Autodesk Inventor part; units mm, degrees
(part 2 of 3)
  line L293 (-765.7551, -84.2338) -> (-765.6693, -83.5816) projected
  line L294 (-765.6693, -83.5816) -> (-765.4175, -82.9738) projected
  line L295 (-765.4175, -82.9738) -> (-765.017, -82.4519) projected
  line L296 (-765.017, -82.4519) -> (-764.4951, -82.0514) projected
  line L297 (-764.4951, -82.0514) -> (-763.8874, -81.7997) projected
  line L298 (-763.8874, -81.7997) -> (-763.2351, -81.7138) projected
  line L299 (-763.2351, -81.7138) -> (-762.5829, -81.7997) projected
  line L300 (-762.5829, -81.7997) -> (-761.9751, -82.0514) projected
  line L301 (-761.9751, -82.0514) -> (-761.4532, -82.4519) projected
  line L302 (-761.4532, -82.4519) -> (-761.0528, -82.9738) projected
  line L303 (-691.0528, -27.9738) -> (-690.801, -28.5816) projected
  line L304 (-690.801, -28.5816) -> (-690.7151, -29.2338) projected
  line L305 (-690.7151, -29.2338) -> (-690.801, -29.886) projected
  line L306 (-690.801, -29.886) -> (-691.0528, -30.4938) projected
  line L307 (-691.0528, -30.4938) -> (-691.4532, -31.0157) projected
  line L308 (-691.4532, -31.0157) -> (-691.9751, -31.4162) projected
  line L309 (-691.9751, -31.4162) -> (-692.5829, -31.6679) projected
  line L310 (-692.5829, -31.6679) -> (-693.2351, -31.7538) projected
  line L311 (-693.2351, -31.7538) -> (-693.8874, -31.6679) projected
  line L312 (-693.8874, -31.6679) -> (-694.4951, -31.4162) projected
  line L313 (-694.4951, -31.4162) -> (-695.0171, -31.0157) projected
  line L314 (-695.0171, -31.0157) -> (-695.4175, -30.4938) projected
  line L315 (-695.4175, -30.4938) -> (-695.6693, -29.886) projected
  line L316 (-695.6693, -29.886) -> (-695.7551, -29.2338) projected
  line L317 (-695.7551, -29.2338) -> (-695.6693, -28.5816) projected
  line L318 (-695.6693, -28.5816) -> (-695.4175, -27.9738) projected
  line L319 (-695.4175, -27.9738) -> (-695.0171, -27.4519) projected
  line L320 (-695.0171, -27.4519) -> (-694.4951, -27.0514) projected
  line L321 (-694.4951, -27.0514) -> (-693.8874, -26.7997) projected
  line L322 (-693.8874, -26.7997) -> (-693.2351, -26.7138) projected
  line L323 (-693.2351, -26.7138) -> (-692.5829, -26.7997) projected
  line L324 (-692.5829, -26.7997) -> (-691.9751, -27.0514) projected
  line L325 (-691.9751, -27.0514) -> (-691.4532, -27.4519) projected
  line L326 (-691.4532, -27.4519) -> (-691.0528, -27.9738) projected
  line L327 (-691.0528, -660.4938) -> (-691.4532, -661.0157) projected
  line L328 (-691.4532, -661.0157) -> (-691.9751, -661.4162) projected
  line L329 (-691.9751, -661.4162) -> (-692.5829, -661.6679) projected
  line L330 (-692.5829, -661.6679) -> (-693.2351, -661.7538) projected
  line L331 (-693.2351, -661.7538) -> (-693.8874, -661.6679) projected
  line L332 (-693.8874, -661.6679) -> (-694.4951, -661.4162) projected
  line L333 (-694.4951, -661.4162) -> (-695.0171, -661.0157) projected
  line L334 (-695.0171, -661.0157) -> (-695.4175, -660.4938) projected
  line L335 (-695.4175, -660.4938) -> (-695.6693, -659.886) projected
  line L336 (-695.6693, -659.886) -> (-695.7551, -659.2338) projected
  line L337 (-695.7551, -659.2338) -> (-695.6693, -658.5816) projected
  line L338 (-695.6693, -658.5816) -> (-695.4175, -657.9738) projected
  line L339 (-695.4175, -657.9738) -> (-695.0171, -657.4519) projected
  line L340 (-695.0171, -657.4519) -> (-694.4951, -657.0514) projected
  line L341 (-694.4951, -657.0514) -> (-693.8874, -656.7997) projected
  line L342 (-693.8874, -656.7997) -> (-693.2351, -656.7138) projected
  line L343 (-693.2351, -656.7138) -> (-692.5829, -656.7997) projected
  line L344 (-692.5829, -656.7997) -> (-691.9751, -657.0514) projected
  line L345 (-691.9751, -657.0514) -> (-691.4532, -657.4519) projected
  line L346 (-691.4532, -657.4519) -> (-691.0528, -657.9738) projected
  line L347 (-691.0528, -657.9738) -> (-690.801, -658.5816) projected
  line L348 (-690.801, -658.5816) -> (-690.7151, -659.2338) projected
  line L349 (-690.7151, -659.2338) -> (-690.801, -659.886) projected
  line L350 (-690.801, -659.886) -> (-691.0528, -660.4938) projected
  line L351 (-761.0528, -27.9738) -> (-760.801, -28.5816) projected
  line L352 (-760.801, -28.5816) -> (-760.7151, -29.2338) projected
  line L353 (-760.7151, -29.2338) -> (-760.801, -29.886) projected
  line L354 (-760.801, -29.886) -> (-761.0528, -30.4938) projected
  line L355 (-761.0528, -30.4938) -> (-761.4532, -31.0157) projected
  line L356 (-761.4532, -31.0157) -> (-761.9751, -31.4162) projected
  line L357 (-761.9751, -31.4162) -> (-762.5829, -31.6679) projected
  line L358 (-762.5829, -31.6679) -> (-763.2351, -31.7538) projected
  line L359 (-763.2351, -31.7538) -> (-763.8874, -31.6679) projected
  line L360 (-763.8874, -31.6679) -> (-764.4951, -31.4162) projected
  line L361 (-764.4951, -31.4162) -> (-765.017, -31.0157) projected
  line L362 (-765.017, -31.0157) -> (-765.4175, -30.4938) projected
  line L363 (-765.4175, -30.4938) -> (-765.6693, -29.886) projected
  line L364 (-765.6693, -29.886) -> (-765.7551, -29.2338) projected
  line L365 (-765.7551, -29.2338) -> (-765.6693, -28.5816) projected
  line L366 (-765.6693, -28.5816) -> (-765.4175, -27.9738) projected
  line L367 (-765.4175, -27.9738) -> (-765.017, -27.4519) projected
  line L368 (-765.017, -27.4519) -> (-764.4951, -27.0514) projected
  line L369 (-764.4951, -27.0514) -> (-763.8874, -26.7997) projected
  line L370 (-763.8874, -26.7997) -> (-763.2351, -26.7138) projected
  line L371 (-763.2351, -26.7138) -> (-762.5829, -26.7997) projected
  line L372 (-762.5829, -26.7997) -> (-761.9751, -27.0514) projected
  line L373 (-761.9751, -27.0514) -> (-761.4532, -27.4519) projected
  line L374 (-761.4532, -27.4519) -> (-761.0528, -27.9738) projected
  line L375 (-761.0528, -657.9738) -> (-760.801, -658.5816) projected
  line L376 (-760.801, -658.5816) -> (-760.7151, -659.2338) projected
  line L377 (-760.7151, -659.2338) -> (-760.801, -659.886) projected
  line L378 (-760.801, -659.886) -> (-761.0528, -660.4938) projected
  line L379 (-761.0528, -660.4938) -> (-761.4532, -661.0157) projected
  line L380 (-761.4532, -661.0157) -> (-761.9751, -661.4162) projected
  line L381 (-761.9751, -661.4162) -> (-762.5829, -661.6679) projected
  line L382 (-762.5829, -661.6679) -> (-763.2351, -661.7538) projected
  line L383 (-763.2351, -661.7538) -> (-763.8874, -661.6679) projected
  line L384 (-763.8874, -661.6679) -> (-764.4951, -661.4162) projected
  line L385 (-764.4951, -661.4162) -> (-765.017, -661.0157) projected
  line L386 (-765.017, -661.0157) -> (-765.4175, -660.4938) projected
  line L387 (-765.4175, -660.4938) -> (-765.6693, -659.886) projected
  line L388 (-765.6693, -659.886) -> (-765.7551, -659.2338) projected
  line L389 (-765.7551, -659.2338) -> (-765.6693, -658.5816) projected
  line L390 (-765.6693, -658.5816) -> (-765.4175, -657.9738) projected
  line L391 (-765.4175, -657.9738) -> (-765.017, -657.4519) projected
  line L392 (-765.017, -657.4519) -> (-764.4951, -657.0514) projected
  line L393 (-764.4951, -657.0514) -> (-763.8874, -656.7997) projected
  line L394 (-763.8874, -656.7997) -> (-763.2351, -656.7138) projected
  line L395 (-763.2351, -656.7138) -> (-762.5829, -656.7997) projected
  line L396 (-762.5829, -656.7997) -> (-761.9751, -657.0514) projected
  line L397 (-761.9751, -657.0514) -> (-761.4532, -657.4519) projected
  line L398 (-761.4532, -657.4519) -> (-761.0528, -657.9738) projected
  line L399 (-640.017, -661.0157) -> (-640.4175, -660.4938) projected
  line L400 (-640.4175, -660.4938) -> (-640.6693, -659.886) projected
  line L401 (-640.6693, -659.886) -> (-640.7551, -659.2338) projected
  line L402 (-640.7551, -659.2338) -> (-640.6693, -658.5816) projected
  line L403 (-640.6693, -658.5816) -> (-640.4175, -657.9738) projected
  line L404 (-640.4175, -657.9738) -> (-640.017, -657.4519) projected
  line L405 (-640.017, -657.4519) -> (-639.4951, -657.0514) projected
  line L406 (-639.4951, -657.0514) -> (-638.8874, -656.7997) projected
  line L407 (-638.8874, -656.7997) -> (-638.2351, -656.7138) projected
  line L408 (-638.2351, -656.7138) -> (-637.5829, -656.7997) projected
  line L409 (-637.5829, -656.7997) -> (-636.9751, -657.0514) projected
  line L410 (-636.9751, -657.0514) -> (-636.4532, -657.4519) projected
  line L411 (-636.4532, -657.4519) -> (-636.0528, -657.9738) projected
  line L412 (-636.0528, -657.9738) -> (-635.801, -658.5816) projected
  line L413 (-635.801, -658.5816) -> (-635.7152, -659.2338) projected
  line L414 (-635.7152, -659.2338) -> (-635.801, -659.886) projected
  line L415 (-635.801, -659.886) -> (-636.0528, -660.4938) projected
  line L416 (-636.0528, -660.4938) -> (-636.4532, -661.0157) projected
  line L417 (-636.4532, -661.0157) -> (-636.9751, -661.4162) projected
  line L418 (-636.9751, -661.4162) -> (-637.5829, -661.6679) projected
  line L419 (-637.5829, -661.6679) -> (-638.2351, -661.7538) projected
  line L420 (-638.2351, -661.7538) -> (-638.8874, -661.6679) projected
  line L421 (-638.8874, -661.6679) -> (-639.4951, -661.4162) projected
  line L422 (-639.4951, -661.4162) -> (-640.017, -661.0157) projected
  line L423 (-636.0528, -27.9738) -> (-635.801, -28.5816) projected
  line L424 (-635.801, -28.5816) -> (-635.7152, -29.2338) projected
  line L425 (-635.7152, -29.2338) -> (-635.801, -29.886) projected
  line L426 (-635.801, -29.886) -> (-636.0528, -30.4938) projected
  line L427 (-636.0528, -30.4938) -> (-636.4532, -31.0157) projected
  line L428 (-636.4532, -31.0157) -> (-636.9751, -31.4162) projected
  line L429 (-636.9751, -31.4162) -> (-637.5829, -31.6679) projected
  line L430 (-637.5829, -31.6679) -> (-638.2351, -31.7538) projected
  line L431 (-638.2351, -31.7538) -> (-638.8874, -31.6679) projected
  line L432 (-638.8874, -31.6679) -> (-639.4951, -31.4162) projected
  line L433 (-639.4951, -31.4162) -> (-640.017, -31.0157) projected
  line L434 (-640.017, -31.0157) -> (-640.4175, -30.4938) projected
  line L435 (-640.4175, -30.4938) -> (-640.6693, -29.886) projected
  line L436 (-640.6693, -29.886) -> (-640.7551, -29.2338) projected
  line L437 (-640.7551, -29.2338) -> (-640.6693, -28.5816) projected
  line L438 (-640.6693, -28.5816) -> (-640.4175, -27.9738) projected
  line L439 (-640.4175, -27.9738) -> (-640.017, -27.4519) projected
  line L440 (-640.017, -27.4519) -> (-639.4951, -27.0514) projected
  line L441 (-639.4951, -27.0514) -> (-638.8874, -26.7997) projected
  line L442 (-638.8874, -26.7997) -> (-638.2351, -26.7138) projected
  line L443 (-638.2351, -26.7138) -> (-637.5829, -26.7997) projected
  line L444 (-637.5829, -26.7997) -> (-636.9751, -27.0514) projected
  line L445 (-636.9751, -27.0514) -> (-636.4532, -27.4519) projected
  line L446 (-636.4532, -27.4519) -> (-636.0528, -27.9738) projected
  line L447 (-727.2351, -219.1338) -> (-726.821, -219.1883) projected
  line L448 (-726.821, -219.1883) -> (-726.4351, -219.3482) projected
  line L449 (-726.4351, -219.3482) -> (-726.1038, -219.6024) projected
  line L450 (-726.1038, -219.6024) -> (-725.8495, -219.9338) projected
  line L451 (-725.8495, -219.9338) -> (-725.6896, -220.3197) projected
  line L452 (-725.6896, -220.3197) -> (-725.6351, -220.7338) projected
  line L453 (-725.6351, -220.7338) -> (-725.6896, -221.1479) projected
  line L454 (-725.6896, -221.1479) -> (-725.8495, -221.5338) projected
  line L455 (-725.8495, -221.5338) -> (-726.1038, -221.8651) projected
  line L456 (-726.1038, -221.8651) -> (-726.4351, -222.1194) projected
  line L457 (-726.4351, -222.1194) -> (-726.821, -222.2793) projected
  line L458 (-726.821, -222.2793) -> (-727.2351, -222.3338) projected
  line L459 (-727.2351, -222.3338) -> (-727.6493, -222.2793) projected
  line L460 (-727.6493, -222.2793) -> (-728.0351, -222.1194) projected
  line L461 (-728.0351, -222.1194) -> (-728.3665, -221.8651) projected
  line L462 (-728.3665, -221.8651) -> (-728.6208, -221.5338) projected
  line L463 (-728.6208, -221.5338) -> (-728.7806, -221.1479) projected
  line L464 (-728.7806, -221.1479) -> (-728.8351, -220.7338) projected
  line L465 (-728.8351, -220.7338) -> (-728.7806, -220.3197) projected
  line L466 (-728.7806, -220.3197) -> (-728.6208, -219.9338) projected
  line L467 (-728.6208, -219.9338) -> (-728.3665, -219.6024) projected
  line L468 (-728.3665, -219.6024) -> (-728.0351, -219.3482) projected
  line L469 (-728.0351, -219.3482) -> (-727.6493, -219.1883) projected
  line L470 (-727.6493, -219.1883) -> (-727.2351, -219.1338) projected
  line L471 (-678.2351, -604.2338) -> (-611.7707, -670.6983) projected
  line L472 (-678.2351, -84.2338) -> (-678.2351, -604.2338) projected
  line L473 (-611.7707, -17.7693) -> (-678.2351, -84.2338) projected
  line L474 (-611.5131, -17.4555) -> (-611.7707, -17.7693) projected
  line L475 (-611.3217, -17.0974) -> (-611.5131, -17.4555) projected
  line L476 (-611.2039, -16.7089) -> (-611.3217, -17.0974) projected
  line L477 (-611.1641, -16.3049) -> (-611.2039, -16.7089) projected
  line L478 (-611.2039, -15.9008) -> (-611.1641, -16.3049) projected
  line L479 (-611.3217, -15.5123) -> (-611.2039, -15.9008) projected
  line L480 (-611.5131, -15.1542) -> (-611.3217, -15.5123) projected
  line L481 (-611.7707, -14.8404) -> (-611.5131, -15.1542) projected
  line L482 (-612.0845, -14.5828) -> (-611.7707, -14.8404) projected
  line L483 (-612.4426, -14.3915) -> (-612.0845, -14.5828) projected
  line L484 (-612.8311, -14.2736) -> (-612.4426, -14.3915) projected
  line L485 (-613.2351, -14.2338) -> (-612.8311, -14.2736) projected
  line L486 (-777.2351, -14.2338) -> (-613.2351, -14.2338) projected
  line L487 (-777.2351, -674.2338) -> (-777.2351, -14.2338) projected
  line L488 (-613.2351, -674.2338) -> (-777.2351, -674.2338) projected
  line L489 (-612.8311, -674.194) -> (-613.2351, -674.2338) projected
  line L490 (-612.4426, -674.0761) -> (-612.8311, -674.194) projected
  line L491 (-612.0845, -673.8848) -> (-612.4426, -674.0761) projected
  line L492 (-611.7707, -673.6272) -> (-612.0845, -673.8848) projected
  line L493 (-611.5131, -673.3134) -> (-611.7707, -673.6272) projected
  line L494 (-611.3217, -672.9553) -> (-611.5131, -673.3134) projected
  line L495 (-611.2039, -672.5668) -> (-611.3217, -672.9553) projected
  line L496 (-611.1641, -672.1627) -> (-611.2039, -672.5668) projected
  line L497 (-611.2039, -671.7587) -> (-611.1641, -672.1627) projected
  line L498 (-611.3217, -671.3702) -> (-611.2039, -671.7587) projected
  line L499 (-611.5131, -671.0121) -> (-611.3217, -671.3702) projected
  line L500 (-611.7707, -670.6983) -> (-611.5131, -671.0121) projected
  line L501 (-747.1924, -48.5812) -> (-747.2351, -49.2338)
  line L502 (-747.2351, -49.2338) -> (-747.2351, -210.2338)
  line L503 (-747.2351, -210.2338) -> (-747.1924, -210.8864)
  line L504 (-747.1924, -210.8864) -> (-747.0648, -211.5279)
  line L505 (-747.0648, -211.5279) -> (-746.8545, -212.1472)
  line L506 (-746.8545, -212.1472) -> (-746.5653, -212.7338)
  line L507 (-746.5653, -212.7338) -> (-746.2019, -213.2776)
  line L508 (-746.2019, -213.2776) -> (-745.7707, -213.7693)
  line L509 (-745.7707, -213.7693) -> (-745.2789, -214.2006)
  line L510 (-745.2789, -214.2006) -> (-744.7351, -214.5639)
  line L511 (-744.7351, -214.5639) -> (-744.1486, -214.8532)
  line L512 (-744.1486, -214.8532) -> (-743.5292, -215.0634)
  line L513 (-743.5292, -215.0634) -> (-742.8878, -215.191)
  line L514 (-742.8878, -215.191) -> (-742.2351, -215.2338)
  line L515 (-742.2351, -215.2338) -> (-713.2351, -215.2338)
  line L516 (-713.2351, -215.2338) -> (-712.5825, -215.191)
  line L517 (-712.5825, -215.191) -> (-711.941, -215.0634)
  line L518 (-711.941, -215.0634) -> (-711.3217, -214.8532)
  line L519 (-711.3217, -214.8532) -> (-710.7351, -214.5639)
  line L520 (-710.7351, -214.5639) -> (-710.1913, -214.2006)
  line L521 (-710.1913, -214.2006) -> (-709.6996, -213.7693)
  line L522 (-709.6996, -213.7693) -> (-709.2684, -213.2776)
  line L523 (-709.2684, -213.2776) -> (-708.905, -212.7338)
  line L524 (-708.905, -212.7338) -> (-708.6157, -212.1472)
  line L525 (-708.6157, -212.1472) -> (-708.4055, -211.5279)
  line L526 (-708.4055, -211.5279) -> (-708.2779, -210.8864)
  line L527 (-708.2779, -210.8864) -> (-708.2351, -210.2338)
  line L528 (-708.2351, -210.2338) -> (-708.2351, -49.2338)
  line L529 (-708.2351, -49.2338) -> (-708.2779, -48.5812)
  line L530 (-708.2779, -48.5812) -> (-708.4055, -47.9397)
  line L531 (-708.4055, -47.9397) -> (-708.6157, -47.3204)
  line L532 (-708.6157, -47.3204) -> (-708.905, -46.7338)
  line L533 (-708.905, -46.7338) -> (-709.2684, -46.19)
  line L534 (-709.2684, -46.19) -> (-709.6996, -45.6983)
  line L535 (-709.6996, -45.6983) -> (-710.1913, -45.267)
  line L536 (-710.1913, -45.267) -> (-710.7351, -44.9037)
  line L537 (-710.7351, -44.9037) -> (-711.3217, -44.6144)
  line L538 (-711.3217, -44.6144) -> (-711.941, -44.4042)
  line L539 (-711.941, -44.4042) -> (-712.5825, -44.2766)
  line L540 (-712.5825, -44.2766) -> (-713.2351, -44.2338)
  line L541 (-713.2351, -44.2338) -> (-742.2351, -44.2338)
  line L542 (-742.2351, -44.2338) -> (-742.8878, -44.2766)
  line L543 (-742.8878, -44.2766) -> (-743.5292, -44.4042)
  line L544 (-743.5292, -44.4042) -> (-744.1486, -44.6144)
  line L545 (-744.1486, -44.6144) -> (-744.7351, -44.9037)
  line L546 (-744.7351, -44.9037) -> (-745.2789, -45.267)
  line L547 (-745.2789, -45.267) -> (-745.7707, -45.6983)
  line L548 (-745.7707, -45.6983) -> (-746.2019, -46.19)
  line L549 (-746.2019, -46.19) -> (-746.5653, -46.7338)
  line L550 (-746.5653, -46.7338) -> (-746.8545, -47.3204)
  line L551 (-746.8545, -47.3204) -> (-747.0648, -47.9397)
  line L552 (-747.0648, -47.9397) -> (-747.1924, -48.5812)
  point P0 (-1999.0141, -29.8543)
  constraints: 210 end point, 52 symmetric about line, 1 horizontal, 1 midpoint
extrude "Extrusion2" cut sketch "Sketch2" against normal blind 3 contours L552 L551 L550 L549 L548 L547 L546 L545 L544 L543 L542 L541 L540 L539 L538 L537 L536 L535 L534 L533 L532 L531 L530 L529 L528 L527 L526 L525 L524 L523 L522 L521 L520 L519 L518 L517 L516 L515 L514 L513 L512 L511 L510 L509 L508 L507 L506 L505 L504 L503 L502 L501
sketch "Sketch3" plane through (-1999.0141, 29.8543, -2600.6334) normal (0, 0, -1) x (-1, 0, 0)
  line L0 (-746.2019, -213.2776) -> (-746.5653, -212.7338) projected
  line L1 (-746.5653, -212.7338) -> (-746.8545, -212.1472) projected
  line L2 (-746.8545, -212.1472) -> (-747.0648, -211.5279) projected
  line L3 (-747.0648, -211.5279) -> (-747.1924, -210.8864) projected
  line L4 (-747.1924, -210.8864) -> (-747.2351, -210.2338) projected
  line L5 (-747.2351, -210.2338) -> (-747.2351, -49.2338) projected
  line L6 (-747.2351, -49.2338) -> (-747.1924, -48.5812) projected
  line L7 (-747.1924, -48.5812) -> (-747.0648, -47.9397) projected
  line L8 (-747.0648, -47.9397) -> (-746.8545, -47.3204) projected
  line L9 (-746.8545, -47.3204) -> (-746.5653, -46.7338) projected
  line L10 (-746.5653, -46.7338) -> (-746.2019, -46.19) projected
  line L11 (-746.2019, -46.19) -> (-745.7707, -45.6983) projected
  line L12 (-745.7707, -45.6983) -> (-745.2789, -45.267) projected
  line L13 (-745.2789, -45.267) -> (-744.7351, -44.9037) projected
  line L14 (-744.7351, -44.9037) -> (-744.1486, -44.6144) projected
  line L15 (-744.1486, -44.6144) -> (-743.5292, -44.4042) projected
  line L16 (-743.5292, -44.4042) -> (-742.8878, -44.2766) projected
  line L17 (-742.8878, -44.2766) -> (-742.2351, -44.2338) projected
  line L18 (-742.2351, -44.2338) -> (-713.2351, -44.2338) projected
  line L19 (-713.2351, -44.2338) -> (-712.5825, -44.2766) projected
  line L20 (-712.5825, -44.2766) -> (-711.941, -44.4042) projected
  line L21 (-711.941, -44.4042) -> (-711.3217, -44.6144) projected
  line L22 (-711.3217, -44.6144) -> (-710.7351, -44.9037) projected
  line L23 (-710.7351, -44.9037) -> (-710.1913, -45.267) projected
  line L24 (-710.1913, -45.267) -> (-709.6996, -45.6983) projected
  line L25 (-709.6996, -45.6983) -> (-709.2684, -46.19) projected
  line L26 (-709.2684, -46.19) -> (-708.905, -46.7338) projected
  line L27 (-708.905, -46.7338) -> (-708.6157, -47.3204) projected
  line L28 (-708.6157, -47.3204) -> (-708.4055, -47.9397) projected
  line L29 (-708.4055, -47.9397) -> (-708.2779, -48.5812) projected
  line L30 (-708.2779, -48.5812) -> (-708.2351, -49.2338) projected
  line L31 (-708.2351, -49.2338) -> (-708.2351, -210.2338) projected
  line L32 (-708.2351, -210.2338) -> (-708.2779, -210.8864) projected
  line L33 (-708.2779, -210.8864) -> (-708.4055, -211.5279) projected
  line L34 (-708.4055, -211.5279) -> (-708.6157, -212.1472) projected
  line L35 (-708.6157, -212.1472) -> (-708.905, -212.7338) projected
  line L36 (-708.905, -212.7338) -> (-709.2684, -213.2776) projected
  line L37 (-709.2684, -213.2776) -> (-709.6996, -213.7693) projected
  line L38 (-709.6996, -213.7693) -> (-710.1913, -214.2006) projected
  line L39 (-710.1913, -214.2006) -> (-710.7351, -214.5639) projected
  line L40 (-710.7351, -214.5639) -> (-711.3217, -214.8532) projected
  line L41 (-711.3217, -214.8532) -> (-711.941, -215.0634) projected
  line L42 (-711.941, -215.0634) -> (-712.5825, -215.191) projected
  line L43 (-712.5825, -215.191) -> (-713.2351, -215.2338) projected
  line L44 (-713.2351, -215.2338) -> (-742.2351, -215.2338) projected
  line L45 (-742.2351, -215.2338) -> (-742.8878, -215.191) projected
  line L46 (-742.8878, -215.191) -> (-743.5292, -215.0634) projected
  line L47 (-743.5292, -215.0634) -> (-744.1486, -214.8532) projected
  line L48 (-744.1486, -214.8532) -> (-744.7351, -214.5639) projected
  line L49 (-744.7351, -214.5639) -> (-745.2789, -214.2006) projected
  line L50 (-745.2789, -214.2006) -> (-745.7707, -213.7693) projected
  line L51 (-745.7707, -213.7693) -> (-746.2019, -213.2776) projected
  line L52 (-747.1924, -639.8864) -> (-747.2351, -639.2338) projected
  line L53 (-747.2351, -639.2338) -> (-747.2351, -478.2338) projected
  line L54 (-747.2351, -478.2338) -> (-747.1924, -477.5812) projected
  line L55 (-747.1924, -477.5812) -> (-747.0648, -476.9397) projected
  line L56 (-747.0648, -476.9397) -> (-746.8545, -476.3204) projected
  line L57 (-746.8545, -476.3204) -> (-746.5653, -475.7338) projected
  line L58 (-746.5653, -475.7338) -> (-746.2019, -475.19) projected
  line L59 (-746.2019, -475.19) -> (-745.7707, -474.6983) projected
  line L60 (-745.7707, -474.6983) -> (-745.2789, -474.267) projected
  line L61 (-745.2789, -474.267) -> (-744.7351, -473.9037) projected
  line L62 (-744.7351, -473.9037) -> (-744.1486, -473.6144) projected
  line L63 (-744.1486, -473.6144) -> (-743.5292, -473.4042) projected
  line L64 (-743.5292, -473.4042) -> (-742.8878, -473.2766) projected
  line L65 (-742.8878, -473.2766) -> (-742.2351, -473.2338) projected
  line L66 (-742.2351, -473.2338) -> (-713.2351, -473.2338) projected
  line L67 (-713.2351, -473.2338) -> (-712.5825, -473.2766) projected
  line L68 (-712.5825, -473.2766) -> (-711.941, -473.4042) projected
  line L69 (-711.941, -473.4042) -> (-711.3217, -473.6144) projected
  line L70 (-711.3217, -473.6144) -> (-710.7351, -473.9037) projected
  line L71 (-710.7351, -473.9037) -> (-710.1913, -474.267) projected
  line L72 (-710.1913, -474.267) -> (-709.6996, -474.6983) projected
  line L73 (-709.6996, -474.6983) -> (-709.2684, -475.19) projected
  line L74 (-709.2684, -475.19) -> (-708.905, -475.7338) projected
  line L75 (-708.905, -475.7338) -> (-708.6157, -476.3204) projected
  line L76 (-708.6157, -476.3204) -> (-708.4055, -476.9397) projected
  line L77 (-708.4055, -476.9397) -> (-708.2779, -477.5812) projected
  line L78 (-708.2779, -477.5812) -> (-708.2351, -478.2338) projected
  line L79 (-708.2351, -478.2338) -> (-708.2351, -639.2338) projected
  line L80 (-708.2351, -639.2338) -> (-708.2779, -639.8864) projected
  line L81 (-708.2779, -639.8864) -> (-708.4055, -640.5279) projected
  line L82 (-708.4055, -640.5279) -> (-708.6157, -641.1472) projected
  line L83 (-708.6157, -641.1472) -> (-708.905, -641.7338) projected
  line L84 (-708.905, -641.7338) -> (-709.2684, -642.2776) projected
  line L85 (-709.2684, -642.2776) -> (-709.6996, -642.7693) projected
  line L86 (-709.6996, -642.7693) -> (-710.1913, -643.2006) projected
  line L87 (-710.1913, -643.2006) -> (-710.7351, -643.5639) projected
  line L88 (-710.7351, -643.5639) -> (-711.3217, -643.8532) projected
  line L89 (-711.3217, -643.8532) -> (-711.941, -644.0634) projected
  line L90 (-711.941, -644.0634) -> (-712.5825, -644.191) projected
  line L91 (-712.5825, -644.191) -> (-713.2351, -644.2338) projected
  line L92 (-713.2351, -644.2338) -> (-742.2351, -644.2338) projected
  line L93 (-742.2351, -644.2338) -> (-742.8878, -644.191) projected
  line L94 (-742.8878, -644.191) -> (-743.5292, -644.0634) projected
  line L95 (-743.5292, -644.0634) -> (-744.1486, -643.8532) projected
  line L96 (-744.1486, -643.8532) -> (-744.7351, -643.5639) projected
  line L97 (-744.7351, -643.5639) -> (-745.2789, -643.2006) projected
  line L98 (-745.2789, -643.2006) -> (-745.7707, -642.7693) projected
  line L99 (-745.7707, -642.7693) -> (-746.2019, -642.2776) projected
  line L100 (-746.2019, -642.2776) -> (-746.5653, -641.7338) projected
  line L101 (-746.5653, -641.7338) -> (-746.8545, -641.1472) projected
  line L102 (-746.8545, -641.1472) -> (-747.0648, -640.5279) projected
  line L103 (-747.0648, -640.5279) -> (-747.1924, -639.8864) projected
  line L104 (-719.7244, -222.8338) -> (-719.7244, -219.2338) projected
  line L105 (-719.7244, -219.2338) -> (-713.5244, -219.2338) projected
  line L106 (-713.5244, -219.2338) -> (-713.5244, -222.8338) projected
  line L107 (-713.5244, -222.8338) -> (-719.7244, -222.8338) projected
  line L108 (-734.7244, -219.2338) -> (-734.7244, -222.8338) projected
  line L109 (-734.7244, -222.8338) -> (-740.9244, -222.8338) projected
  line L110 (-740.9244, -222.8338) -> (-740.9244, -219.2338) projected
  line L111 (-740.9244, -219.2338) -> (-734.7244, -219.2338) projected
  line L112 (-691.0528, -342.9738) -> (-690.801, -343.5816) projected
  line L113 (-690.801, -343.5816) -> (-690.7151, -344.2338) projected
  line L114 (-690.7151, -344.2338) -> (-690.801, -344.886) projected
  line L115 (-690.801, -344.886) -> (-691.0528, -345.4938) projected
  line L116 (-691.0528, -345.4938) -> (-691.4532, -346.0157) projected
  line L117 (-691.4532, -346.0157) -> (-691.9751, -346.4162) projected
  line L118 (-691.9751, -346.4162) -> (-692.5829, -346.6679) projected
  line L119 (-692.5829, -346.6679) -> (-693.2351, -346.7538) projected
  line L120 (-693.2351, -346.7538) -> (-693.8874, -346.6679) projected
  line L121 (-693.8874, -346.6679) -> (-694.4951, -346.4162) projected
  line L122 (-694.4951, -346.4162) -> (-695.0171, -346.0157) projected
  line L123 (-695.0171, -346.0157) -> (-695.4175, -345.4938) projected
  line L124 (-695.4175, -345.4938) -> (-695.6693, -344.886) projected
  line L125 (-695.6693, -344.886) -> (-695.7551, -344.2338) projected
  line L126 (-695.7551, -344.2338) -> (-695.6693, -343.5816) projected
  line L127 (-695.6693, -343.5816) -> (-695.4175, -342.9738) projected
  line L128 (-695.4175, -342.9738) -> (-695.0171, -342.4519) projected
  line L129 (-695.0171, -342.4519) -> (-694.4951, -342.0514) projected
  line L130 (-694.4951, -342.0514) -> (-693.8874, -341.7996) projected
  line L131 (-693.8874, -341.7996) -> (-693.2351, -341.7138) projected
  line L132 (-693.2351, -341.7138) -> (-692.5829, -341.7996) projected
  line L133 (-692.5829, -341.7996) -> (-691.9751, -342.0514) projected
  line L134 (-691.9751, -342.0514) -> (-691.4532, -342.4519) projected
  line L135 (-691.4532, -342.4519) -> (-691.0528, -342.9738) projected
  line L136 (-691.4532, -471.4019) -> (-691.0528, -471.9238) projected
  line L137 (-691.0528, -471.9238) -> (-690.801, -472.5316) projected
  line L138 (-690.801, -472.5316) -> (-690.7151, -473.1838) projected
  line L139 (-690.7151, -473.1838) -> (-690.801, -473.836) projected
  line L140 (-690.801, -473.836) -> (-691.0528, -474.4438) projected
  line L141 (-691.0528, -474.4438) -> (-691.4532, -474.9657) projected
  line L142 (-691.4532, -474.9657) -> (-691.9751, -475.3662) projected
  line L143 (-691.9751, -475.3662) -> (-692.5829, -475.6179) projected
  line L144 (-692.5829, -475.6179) -> (-693.2351, -475.7038) projected
  line L145 (-693.2351, -475.7038) -> (-693.8874, -475.6179) projected
  line L146 (-693.8874, -475.6179) -> (-694.4951, -475.3662) projected
  line L147 (-694.4951, -475.3662) -> (-695.0171, -474.9657) projected
  line L148 (-695.0171, -474.9657) -> (-695.4175, -474.4438) projected
  line L149 (-695.4175, -474.4438) -> (-695.6693, -473.836) projected
  line L150 (-695.6693, -473.836) -> (-695.7551, -473.1838) projected
  line L151 (-695.7551, -473.1838) -> (-695.6693, -472.5316) projected
  line L152 (-695.6693, -472.5316) -> (-695.4175, -471.9238) projected
  line L153 (-695.4175, -471.9238) -> (-695.0171, -471.4019) projected
  line L154 (-695.0171, -471.4019) -> (-694.4951, -471.0014) projected
  line L155 (-694.4951, -471.0014) -> (-693.8874, -470.7497) projected
  line L156 (-693.8874, -470.7497) -> (-693.2351, -470.6638) projected
  line L157 (-693.2351, -470.6638) -> (-692.5829, -470.7497) projected
  line L158 (-692.5829, -470.7497) -> (-691.9751, -471.0014) projected
  line L159 (-691.9751, -471.0014) -> (-691.4532, -471.4019) projected
  line L160 (-691.0528, -602.9738) -> (-690.801, -603.5816) projected
  line L161 (-690.801, -603.5816) -> (-690.7151, -604.2338) projected
  line L162 (-690.7151, -604.2338) -> (-690.801, -604.886) projected
  line L163 (-690.801, -604.886) -> (-691.0528, -605.4938) projected
  line L164 (-691.0528, -605.4938) -> (-691.4532, -606.0157) projected
  line L165 (-691.4532, -606.0157) -> (-691.9751, -606.4162) projected
  line L166 (-691.9751, -606.4162) -> (-692.5829, -606.6679) projected
  line L167 (-692.5829, -606.6679) -> (-693.2351, -606.7538) projected
  line L168 (-693.2351, -606.7538) -> (-693.8874, -606.6679) projected
  line L169 (-693.8874, -606.6679) -> (-694.4951, -606.4162) projected
  line L170 (-694.4951, -606.4162) -> (-695.0171, -606.0157) projected
  line L171 (-695.0171, -606.0157) -> (-695.4175, -605.4938) projected
  line L172 (-695.4175, -605.4938) -> (-695.6693, -604.886) projected
  line L173 (-695.6693, -604.886) -> (-695.7551, -604.2338) projected
  line L174 (-695.7551, -604.2338) -> (-695.6693, -603.5816) projected
  line L175 (-695.6693, -603.5816) -> (-695.4175, -602.9738) projected
  line L176 (-695.4175, -602.9738) -> (-695.0171, -602.4519) projected
  line L177 (-695.0171, -602.4519) -> (-694.4951, -602.0514) projected
  line L178 (-694.4951, -602.0514) -> (-693.8874, -601.7997) projected
  line L179 (-693.8874, -601.7997) -> (-693.2351, -601.7138) projected
  line L180 (-693.2351, -601.7138) -> (-692.5829, -601.7997) projected
  line L181 (-692.5829, -601.7997) -> (-691.9751, -602.0514) projected
  line L182 (-691.9751, -602.0514) -> (-691.4532, -602.4519) projected
  line L183 (-691.4532, -602.4519) -> (-691.0528, -602.9738) projected
  line L184 (-691.0528, -214.0238) -> (-690.801, -214.6316) projected
  line L185 (-690.801, -214.6316) -> (-690.7151, -215.2838) projected
  line L186 (-690.7151, -215.2838) -> (-690.801, -215.936) projected
  line L187 (-690.801, -215.936) -> (-691.0528, -216.5438) projected
  line L188 (-691.0528, -216.5438) -> (-691.4532, -217.0657) projected
  line L189 (-691.4532, -217.0657) -> (-691.9751, -217.4662) projected
  line L190 (-691.9751, -217.4662) -> (-692.5829, -217.7179) projected
  line L191 (-692.5829, -217.7179) -> (-693.2351, -217.8038) projected
  line L192 (-693.2351, -217.8038) -> (-693.8874, -217.7179) projected
  line L193 (-693.8874, -217.7179) -> (-694.4951, -217.4662) projected
  line L194 (-694.4951, -217.4662) -> (-695.0171, -217.0657) projected
  line L195 (-695.0171, -217.0657) -> (-695.4175, -216.5438) projected
  line L196 (-695.4175, -216.5438) -> (-695.6693, -215.936) projected
  line L197 (-695.6693, -215.936) -> (-695.7551, -215.2838) projected
  line L198 (-695.7551, -215.2838) -> (-695.6693, -214.6316) projected
  line L199 (-695.6693, -214.6316) -> (-695.4175, -214.0238) projected
  line L200 (-695.4175, -214.0238) -> (-695.0171, -213.5019) projected
  line L201 (-695.0171, -213.5019) -> (-694.4951, -213.1014) projected
  line L202 (-694.4951, -213.1014) -> (-693.8874, -212.8497) projected
  line L203 (-693.8874, -212.8497) -> (-693.2351, -212.7638) projected
  line L204 (-693.2351, -212.7638) -> (-692.5829, -212.8497) projected
  line L205 (-692.5829, -212.8497) -> (-691.9751, -213.1014) projected
  line L206 (-691.9751, -213.1014) -> (-691.4532, -213.5019) projected
  line L207 (-691.4532, -213.5019) -> (-691.0528, -214.0238) projected
  line L208 (-691.9751, -82.0514) -> (-691.4532, -82.4519) projected
  line L209 (-691.4532, -82.4519) -> (-691.0528, -82.9738) projected
  line L210 (-691.0528, -82.9738) -> (-690.801, -83.5816) projected
  line L211 (-690.801, -83.5816) -> (-690.7151, -84.2338) projected
  line L212 (-690.7151, -84.2338) -> (-690.801, -84.886) projected
  line L213 (-690.801, -84.886) -> (-691.0528, -85.4938) projected
  line L214 (-691.0528, -85.4938) -> (-691.4532, -86.0157) projected
  line L215 (-691.4532, -86.0157) -> (-691.9751, -86.4162) projected
  line L216 (-691.9751, -86.4162) -> (-692.5829, -86.6679) projected
  line L217 (-692.5829, -86.6679) -> (-693.2351, -86.7538) projected
  line L218 (-693.2351, -86.7538) -> (-693.8874, -86.6679) projected
  line L219 (-693.8874, -86.6679) -> (-694.4951, -86.4162) projected
  line L220 (-694.4951, -86.4162) -> (-695.0171, -86.0157) projected
  line L221 (-695.0171, -86.0157) -> (-695.4175, -85.4938) projected
  line L222 (-695.4175, -85.4938) -> (-695.6693, -84.886) projected
  line L223 (-695.6693, -84.886) -> (-695.7551, -84.2338) projected
  line L224 (-695.7551, -84.2338) -> (-695.6693, -83.5816) projected
  line L225 (-695.6693, -83.5816) -> (-695.4175, -82.9738) projected
  line L226 (-695.4175, -82.9738) -> (-695.0171, -82.4519) projected
  line L227 (-695.0171, -82.4519) -> (-694.4951, -82.0514) projected
  line L228 (-694.4951, -82.0514) -> (-693.8874, -81.7997) projected
  line L229 (-693.8874, -81.7997) -> (-693.2351, -81.7138) projected
  line L230 (-693.2351, -81.7138) -> (-692.5829, -81.7997) projected
  line L231 (-692.5829, -81.7997) -> (-691.9751, -82.0514) projected
  line L232 (-765.4175, -345.4938) -> (-765.6693, -344.886) projected
  line L233 (-765.6693, -344.886) -> (-765.7551, -344.2338) projected
  line L234 (-765.7551, -344.2338) -> (-765.6693, -343.5816) projected
  line L235 (-765.6693, -343.5816) -> (-765.4175, -342.9738) projected
  line L236 (-765.4175, -342.9738) -> (-765.017, -342.4519) projected
  line L237 (-765.017, -342.4519) -> (-764.4951, -342.0514) projected
  line L238 (-764.4951, -342.0514) -> (-763.8874, -341.7996) projected
  line L239 (-763.8874, -341.7996) -> (-763.2351, -341.7138) projected
  line L240 (-763.2351, -341.7138) -> (-762.5829, -341.7996) projected
  line L241 (-762.5829, -341.7996) -> (-761.9751, -342.0514) projected
  line L242 (-761.9751, -342.0514) -> (-761.4532, -342.4519) projected
  line L243 (-761.4532, -342.4519) -> (-761.0528, -342.9738) projected
  line L244 (-761.0528, -342.9738) -> (-760.801, -343.5816) projected
  line L245 (-760.801, -343.5816) -> (-760.7151, -344.2338) projected
  line L246 (-760.7151, -344.2338) -> (-760.801, -344.886) projected
  line L247 (-760.801, -344.886) -> (-761.0528, -345.4938) projected
  line L248 (-761.0528, -345.4938) -> (-761.4532, -346.0157) projected
  line L249 (-761.4532, -346.0157) -> (-761.9751, -346.4162) projected
  line L250 (-761.9751, -346.4162) -> (-762.5829, -346.6679) projected
  line L251 (-762.5829, -346.6679) -> (-763.2351, -346.7538) projected
  line L252 (-763.2351, -346.7538) -> (-763.8874, -346.6679) projected
  line L253 (-763.8874, -346.6679) -> (-764.4951, -346.4162) projected
  line L254 (-764.4951, -346.4162) -> (-765.017, -346.0157) projected
  line L255 (-765.017, -346.0157) -> (-765.4175, -345.4938) projected
  line L256 (-761.0528, -471.9238) -> (-760.801, -472.5316) projected
  line L257 (-760.801, -472.5316) -> (-760.7151, -473.1838) projected
  line L258 (-760.7151, -473.1838) -> (-760.801, -473.836) projected
  line L259 (-760.801, -473.836) -> (-761.0528, -474.4438) projected
  line L260 (-761.0528, -474.4438) -> (-761.4532, -474.9657) projected
  line L261 (-761.4532, -474.9657) -> (-761.9751, -475.3662) projected
  line L262 (-761.9751, -475.3662) -> (-762.5829, -475.6179) projected
  line L263 (-762.5829, -475.6179) -> (-763.2351, -475.7038) projected
  line L264 (-763.2351, -475.7038) -> (-763.8874, -475.6179) projected
  line L265 (-763.8874, -475.6179) -> (-764.4951, -475.3662) projected
  line L266 (-764.4951, -475.3662) -> (-765.017, -474.9657) projected
  line L267 (-765.017, -474.9657) -> (-765.4175, -474.4438) projected
  line L268 (-765.4175, -474.4438) -> (-765.6693, -473.836) projected
  line L269 (-765.6693, -473.836) -> (-765.7551, -473.1838) projected
  line L270 (-765.7551, -473.1838) -> (-765.6693, -472.5316) projected
  line L271 (-765.6693, -472.5316) -> (-765.4175, -471.9238) projected
  line L272 (-765.4175, -471.9238) -> (-765.017, -471.4019) projected
  line L273 (-765.017, -471.4019) -> (-764.4951, -471.0014) projected
  line L274 (-764.4951, -471.0014) -> (-763.8874, -470.7497) projected
  line L275 (-763.8874, -470.7497) -> (-763.2351, -470.6638) projected
  line L276 (-763.2351, -470.6638) -> (-762.5829, -470.7497) projected
  line L277 (-762.5829, -470.7497) -> (-761.9751, -471.0014) projected
  line L278 (-761.9751, -471.0014) -> (-761.4532, -471.4019) projected
  line L279 (-761.4532, -471.4019) -> (-761.0528, -471.9238) projected
  line L280 (-765.4175, -605.4938) -> (-765.6693, -604.886) projected
  line L281 (-765.6693, -604.886) -> (-765.7551, -604.2338) projected
  line L282 (-765.7551, -604.2338) -> (-765.6693, -603.5816) projected
  line L283 (-765.6693, -603.5816) -> (-765.4175, -602.9738) projected
  line L284 (-765.4175, -602.9738) -> (-765.017, -602.4519) projected
  line L285 (-765.017, -602.4519) -> (-764.4951, -602.0514) projected
  line L286 (-764.4951, -602.0514) -> (-763.8874, -601.7997) projected
  line L287 (-763.8874, -601.7997) -> (-763.2351, -601.7138) projected
  line L288 (-763.2351, -601.7138) -> (-762.5829, -601.7997) projected
  line L289 (-762.5829, -601.7997) -> (-761.9751, -602.0514) projected
  line L290 (-761.9751, -602.0514) -> (-761.4532, -602.4519) projected
  line L291 (-761.4532, -602.4519) -> (-761.0528, -602.9738) projected
  line L292 (-761.0528, -602.9738) -> (-760.801, -603.5816) projected
  line L293 (-760.801, -603.5816) -> (-760.7151, -604.2338) projected
  line L294 (-760.7151, -604.2338) -> (-760.801, -604.886) projected
  line L295 (-760.801, -604.886) -> (-761.0528, -605.4938) projected
  line L296 (-761.0528, -605.4938) -> (-761.4532, -606.0157) projected
  line L297 (-761.4532, -606.0157) -> (-761.9751, -606.4162) projected
  line L298 (-761.9751, -606.4162) -> (-762.5829, -606.6679) projected
  line L299 (-762.5829, -606.6679) -> (-763.2351, -606.7538) projected
  line L300 (-763.2351, -606.7538) -> (-763.8874, -606.6679) projected
  line L301 (-763.8874, -606.6679) -> (-764.4951, -606.4162) projected
  line L302 (-764.4951, -606.4162) -> (-765.017, -606.0157) projected
  line L303 (-765.017, -606.0157) -> (-765.4175, -605.4938) projected
  line L304 (-761.4532, -213.5019) -> (-761.0528, -214.0238) projected
  line L305 (-761.0528, -214.0238) -> (-760.801, -214.6316) projected
  line L306 (-760.801, -214.6316) -> (-760.7151, -215.2838) projected
  line L307 (-760.7151, -215.2838) -> (-760.801, -215.936) projected
  line L308 (-760.801, -215.936) -> (-761.0528, -216.5438) projected
  line L309 (-761.0528, -216.5438) -> (-761.4532, -217.0657) projected
  line L310 (-761.4532, -217.0657) -> (-761.9751, -217.4662) projected
  line L311 (-761.9751, -217.4662) -> (-762.5829, -217.7179) projected
  line L312 (-762.5829, -217.7179) -> (-763.2351, -217.8038) projected
  line L313 (-763.2351, -217.8038) -> (-763.8874, -217.7179) projected
  line L314 (-763.8874, -217.7179) -> (-764.4951, -217.4662) projected
  line L315 (-764.4951, -217.4662) -> (-765.017, -217.0657) projected
  line L316 (-765.017, -217.0657) -> (-765.4175, -216.5438) projected
  line L317 (-765.4175, -216.5438) -> (-765.6693, -215.936) projected
  line L318 (-765.6693, -215.936) -> (-765.7551, -215.2838) projected
  line L319 (-765.7551, -215.2838) -> (-765.6693, -214.6316) projected
  line L320 (-765.6693, -214.6316) -> (-765.4175, -214.0238) projected
  line L321 (-765.4175, -214.0238) -> (-765.017, -213.5019) projected
  line L322 (-765.017, -213.5019) -> (-764.4951, -213.1014) projected
  line L323 (-764.4951, -213.1014) -> (-763.8874, -212.8497) projected
  line L324 (-763.8874, -212.8497) -> (-763.2351, -212.7638) projected
  line L325 (-763.2351, -212.7638) -> (-762.5829, -212.8497) projected
  line L326 (-762.5829, -212.8497) -> (-761.9751, -213.1014) projected
  line L327 (-761.9751, -213.1014) -> (-761.4532, -213.5019) projected
  line L328 (-761.0528, -82.9738) -> (-760.801, -83.5816) projected
  line L329 (-760.801, -83.5816) -> (-760.7151, -84.2338) projected
  line L330 (-760.7151, -84.2338) -> (-760.801, -84.886) projected
  line L331 (-760.801, -84.886) -> (-761.0528, -85.4938) projected
  line L332 (-761.0528, -85.4938) -> (-761.4532, -86.0157) projected
  line L333 (-761.4532, -86.0157) -> (-761.9751, -86.4162) projected
  line L334 (-761.9751, -86.4162) -> (-762.5829, -86.6679) projected
  line L335 (-762.5829, -86.6679) -> (-763.2351, -86.7538) projected
  line L336 (-763.2351, -86.7538) -> (-763.8874, -86.6679) projected
  line L337 (-763.8874, -86.6679) -> (-764.4951, -86.4162) projected
  line L338 (-764.4951, -86.4162) -> (-765.017, -86.0157) projected
  line L339 (-765.017, -86.0157) -> (-765.4175, -85.4938) projected
  line L340 (-765.4175, -85.4938) -> (-765.6693, -84.886) projected
  line L341 (-765.6693, -84.886) -> (-765.7551, -84.2338) projected
  line L342 (-765.7551, -84.2338) -> (-765.6693, -83.5816) projected
  line L343 (-765.6693, -83.5816) -> (-765.4175, -82.9738) projected
  line L344 (-765.4175, -82.9738) -> (-765.017, -82.4519) projected
  line L345 (-765.017, -82.4519) -> (-764.4951, -82.0514) projected
  line L346 (-764.4951, -82.0514) -> (-763.8874, -81.7997) projected
  line L347 (-763.8874, -81.7997) -> (-763.2351, -81.7138) projected
  line L348 (-763.2351, -81.7138) -> (-762.5829, -81.7997) projected
  line L349 (-762.5829, -81.7997) -> (-761.9751, -82.0514) projected
  line L350 (-761.9751, -82.0514) -> (-761.4532, -82.4519) projected
  line L351 (-761.4532, -82.4519) -> (-761.0528, -82.9738) projected
  line L352 (-691.0528, -27.9738) -> (-690.801, -28.5816) projected
  line L353 (-690.801, -28.5816) -> (-690.7151, -29.2338) projected
  line L354 (-690.7151, -29.2338) -> (-690.801, -29.886) projected
  line L355 (-690.801, -29.886) -> (-691.0528, -30.4938) projected
  line L356 (-691.0528, -30.4938) -> (-691.4532, -31.0157) projected
  line L357 (-691.4532, -31.0157) -> (-691.9751, -31.4162) projected
  line L358 (-691.9751, -31.4162) -> (-692.5829, -31.6679) projected
  line L359 (-692.5829, -31.6679) -> (-693.2351, -31.7538) projected
  line L360 (-693.2351, -31.7538) -> (-693.8874, -31.6679) projected
  line L361 (-693.8874, -31.6679) -> (-694.4951, -31.4162) projected
  line L362 (-694.4951, -31.4162) -> (-695.0171, -31.0157) projected
  line L363 (-695.0171, -31.0157) -> (-695.4175, -30.4938) projected
  line L364 (-695.4175, -30.4938) -> (-695.6693, -29.886) projected
  line L365 (-695.6693, -29.886) -> (-695.7551, -29.2338) projected
  line L366 (-695.7551, -29.2338) -> (-695.6693, -28.5816) projected
  line L367 (-695.6693, -28.5816) -> (-695.4175, -27.9738) projected
  line L368 (-695.4175, -27.9738) -> (-695.0171, -27.4519) projected
  line L369 (-695.0171, -27.4519) -> (-694.4951, -27.0514) projected
  line L370 (-694.4951, -27.0514) -> (-693.8874, -26.7997) projected
  line L371 (-693.8874, -26.7997) -> (-693.2351, -26.7138) projected
  line L372 (-693.2351, -26.7138) -> (-692.5829, -26.7997) projected
  line L373 (-692.5829, -26.7997) -> (-691.9751, -27.0514) projected
  line L374 (-691.9751, -27.0514) -> (-691.4532, -27.4519) projected
  line L375 (-691.4532, -27.4519) -> (-691.0528, -27.9738) projected
  line L376 (-691.0528, -660.4938) -> (-691.4532, -661.0157) projected
  line L377 (-691.4532, -661.0157) -> (-691.9751, -661.4162) projected
  line L378 (-691.9751, -661.4162) -> (-692.5829, -661.6679) projected
  line L379 (-692.5829, -661.6679) -> (-693.2351, -661.7538) projected
  line L380 (-693.2351, -661.7538) -> (-693.8874, -661.6679) projected
  line L381 (-693.8874, -661.6679) -> (-694.4951, -661.4162) projected
  line L382 (-694.4951, -661.4162) -> (-695.0171, -661.0157) projected
  line L383 (-695.0171, -661.0157) -> (-695.4175, -660.4938) projected
  line L384 (-695.4175, -660.4938) -> (-695.6693, -659.886) projected
  line L385 (-695.6693, -659.886) -> (-695.7551, -659.2338) projected
  line L386 (-695.7551, -659.2338) -> (-695.6693, -658.5816) projected
  line L387 (-695.6693, -658.5816) -> (-695.4175, -657.9738) projected
  line L388 (-695.4175, -657.9738) -> (-695.0171, -657.4519) projected
  line L389 (-695.0171, -657.4519) -> (-694.4951, -657.0514) projected
  line L390 (-694.4951, -657.0514) -> (-693.8874, -656.7997) projected
  line L391 (-693.8874, -656.7997) -> (-693.2351, -656.7138) projected
  line L392 (-693.2351, -656.7138) -> (-692.5829, -656.7997) projected
  line L393 (-692.5829, -656.7997) -> (-691.9751, -657.0514) projected
  line L394 (-691.9751, -657.0514) -> (-691.4532, -657.4519) projected
  line L395 (-691.4532, -657.4519) -> (-691.0528, -657.9738) projected
  line L396 (-691.0528, -657.9738) -> (-690.801, -658.5816) projected
  line L397 (-690.801, -658.5816) -> (-690.7151, -659.2338) projected
  line L398 (-690.7151, -659.2338) -> (-690.801, -659.886) projected
  line L399 (-690.801, -659.886) -> (-691.0528, -660.4938) projected
  line L400 (-761.0528, -27.9738) -> (-760.801, -28.5816) projected
  line L401 (-760.801, -28.5816) -> (-760.7151, -29.2338) projected
  line L402 (-760.7151, -29.2338) -> (-760.801, -29.886) projected
  line L403 (-760.801, -29.886) -> (-761.0528, -30.4938) projected
  line L404 (-761.0528, -30.4938) -> (-761.4532, -31.0157) projected
  line L405 (-761.4532, -31.0157) -> (-761.9751, -31.4162) projected
  line L406 (-761.9751, -31.4162) -> (-762.5829, -31.6679) projected
  line L407 (-762.5829, -31.6679) -> (-763.2351, -31.7538) projected
  line L408 (-763.2351, -31.7538) -> (-763.8874, -31.6679) projected
  line L409 (-763.8874, -31.6679) -> (-764.4951, -31.4162) projected
  line L410 (-764.4951, -31.4162) -> (-765.017, -31.0157) projected
  line L411 (-765.017, -31.0157) -> (-765.4175, -30.4938) projected
  line L412 (-765.4175, -30.4938) -> (-765.6693, -29.886) projected
  line L413 (-765.6693, -29.886) -> (-765.7551, -29.2338) projected
  line L414 (-765.7551, -29.2338) -> (-765.6693, -28.5816) projected
  line L415 (-765.6693, -28.5816) -> (-765.4175, -27.9738) projected
  line L416 (-765.4175, -27.9738) -> (-765.017, -27.4519) projected
  line L417 (-765.017, -27.4519) -> (-764.4951, -27.0514) projected
  line L418 (-764.4951, -27.0514) -> (-763.8874, -26.7997) projected
  line L419 (-763.8874, -26.7997) -> (-763.2351, -26.7138) projected
  line L420 (-763.2351, -26.7138) -> (-762.5829, -26.7997) projected
  line L421 (-762.5829, -26.7997) -> (-761.9751, -27.0514) projected
  line L422 (-761.9751, -27.0514) -> (-761.4532, -27.4519) projected
  line L423 (-761.4532, -27.4519) -> (-761.0528, -27.9738) projected
  line L424 (-761.0528, -657.9738) -> (-760.801, -658.5816) projected
  line L425 (-760.801, -658.5816) -> (-760.7151, -659.2338) projected
  line L426 (-760.7151, -659.2338) -> (-760.801, -659.886) projected
  line L427 (-760.801, -659.886) -> (-761.0528, -660.4938) projected
  line L428 (-761.0528, -660.4938) -> (-761.4532, -661.0157) projected
  line L429 (-761.4532, -661.0157) -> (-761.9751, -661.4162) projected
  line L430 (-761.9751, -661.4162) -> (-762.5829, -661.6679) projected
  line L431 (-762.5829, -661.6679) -> (-763.2351, -661.7538) projected
  line L432 (-763.2351, -661.7538) -> (-763.8874, -661.6679) projected
  line L433 (-763.8874, -661.6679) -> (-764.4951, -661.4162) projected
  line L434 (-764.4951, -661.4162) -> (-765.017, -661.0157) projected
  line L435 (-765.017, -661.0157) -> (-765.4175, -660.4938) projected
  line L436 (-765.4175, -660.4938) -> (-765.6693, -659.886) projected
  line L437 (-765.6693, -659.886) -> (-765.7551, -659.2338) projected
  line L438 (-765.7551, -659.2338) -> (-765.6693, -658.5816) projected
  line L439 (-765.6693, -658.5816) -> (-765.4175, -657.9738) projected
  line L440 (-765.4175, -657.9738) -> (-765.017, -657.4519) projected
  line L441 (-765.017, -657.4519) -> (-764.4951, -657.0514) projected
  line L442 (-764.4951, -657.0514) -> (-763.8874, -656.7997) projected
  line L443 (-763.8874, -656.7997) -> (-763.2351, -656.7138) projected
  line L444 (-763.2351, -656.7138) -> (-762.5829, -656.7997) projected
  line L445 (-762.5829, -656.7997) -> (-761.9751, -657.0514) projected
  line L446 (-761.9751, -657.0514) -> (-761.4532, -657.4519) projected
  line L447 (-761.4532, -657.4519) -> (-761.0528, -657.9738) projected
  line L448 (-640.017, -661.0157) -> (-640.4175, -660.4938) projected
  line L449 (-640.4175, -660.4938) -> (-640.6693, -659.886) projected
  line L450 (-640.6693, -659.886) -> (-640.7551, -659.2338) projected
  line L451 (-640.7551, -659.2338) -> (-640.6693, -658.5816) projected
  line L452 (-640.6693, -658.5816) -> (-640.4175, -657.9738) projected
  line L453 (-640.4175, -657.9738) -> (-640.017, -657.4519) projected
  line L454 (-640.017, -657.4519) -> (-639.4951, -657.0514) projected
  line L455 (-639.4951, -657.0514) -> (-638.8874, -656.7997) projected
  line L456 (-638.8874, -656.7997) -> (-638.2351, -656.7138) projected
  line L457 (-638.2351, -656.7138) -> (-637.5829, -656.7997) projected
  line L458 (-637.5829, -656.7997) -> (-636.9751, -657.0514) projected
  line L459 (-636.9751, -657.0514) -> (-636.4532, -657.4519) projected
  line L460 (-636.4532, -657.4519) -> (-636.0528, -657.9738) projected
  line L461 (-636.0528, -657.9738) -> (-635.801, -658.5816) projected
  line L462 (-635.801, -658.5816) -> (-635.7152, -659.2338) projected
  line L463 (-635.7152, -659.2338) -> (-635.801, -659.886) projected
  line L464 (-635.801, -659.886) -> (-636.0528, -660.4938) projected
  line L465 (-636.0528, -660.4938) -> (-636.4532, -661.0157) projected
  line L466 (-636.4532, -661.0157) -> (-636.9751, -661.4162) projected
  line L467 (-636.9751, -661.4162) -> (-637.5829, -661.6679) projected
  line L468 (-637.5829, -661.6679) -> (-638.2351, -661.7538) projected
  line L469 (-638.2351, -661.7538) -> (-638.8874, -661.6679) projected
  line L470 (-638.8874, -661.6679) -> (-639.4951, -661.4162) projected
  line L471 (-639.4951, -661.4162) -> (-640.017, -661.0157) projected
  line L472 (-636.0528, -27.9738) -> (-635.801, -28.5816) projected
  line L473 (-635.801, -28.5816) -> (-635.7152, -29.2338) projected
  line L474 (-635.7152, -29.2338) -> (-635.801, -29.886) projected
  line L475 (-635.801, -29.886) -> (-636.0528, -30.4938) projected
  line L476 (-636.0528, -30.4938) -> (-636.4532, -31.0157) projected
  line L477 (-636.4532, -31.0157) -> (-636.9751, -31.4162) projected
  line L478 (-636.9751, -31.4162) -> (-637.5829, -31.6679) projected
  line L479 (-637.5829, -31.6679) -> (-638.2351, -31.7538) projected
  line L480 (-638.2351, -31.7538) -> (-638.8874, -31.6679) projected
  line L481 (-638.8874, -31.6679) -> (-639.4951, -31.4162) projected
  line L482 (-639.4951, -31.4162) -> (-640.017, -31.0157) projected
  line L483 (-640.017, -31.0157) -> (-640.4175, -30.4938) projected
  line L484 (-640.4175, -30.4938) -> (-640.6693, -29.886) projected
  line L485 (-640.6693, -29.886) -> (-640.7551, -29.2338) projected
  line L486 (-640.7551, -29.2338) -> (-640.6693, -28.5816) projected
  line L487 (-640.6693, -28.5816) -> (-640.4175, -27.9738) projected
  line L488 (-640.4175, -27.9738) -> (-640.017, -27.4519) projected
  line L489 (-640.017, -27.4519) -> (-639.4951, -27.0514) projected
  line L490 (-639.4951, -27.0514) -> (-638.8874, -26.7997) projected
  line L491 (-638.8874, -26.7997) -> (-638.2351, -26.7138) projected
  line L492 (-638.2351, -26.7138) -> (-637.5829, -26.7997) projected
  line L493 (-637.5829, -26.7997) -> (-636.9751, -27.0514) projected
  line L494 (-636.9751, -27.0514) -> (-636.4532, -27.4519) projected
  line L495 (-636.4532, -27.4519) -> (-636.0528, -27.9738) projected
  line L496 (-727.2351, -219.1338) -> (-726.821, -219.1883) projected
  line L497 (-726.821, -219.1883) -> (-726.4351, -219.3482) projected
  line L498 (-726.4351, -219.3482) -> (-726.1038, -219.6024) projected
  line L499 (-726.1038, -219.6024) -> (-725.8495, -219.9338) projected
  line L500 (-725.8495, -219.9338) -> (-725.6896, -220.3197) projected
  line L501 (-725.6896, -220.3197) -> (-725.6351, -220.7338) projected
  line L502 (-725.6351, -220.7338) -> (-725.6896, -221.1479) projected
  line L503 (-725.6896, -221.1479) -> (-725.8495, -221.5338) projected
  line L504 (-725.8495, -221.5338) -> (-726.1038, -221.8651) projected
  line L505 (-726.1038, -221.8651) -> (-726.4351, -222.1194) projected
  line L506 (-726.4351, -222.1194) -> (-726.821, -222.2793) projected
  line L507 (-726.821, -222.2793) -> (-727.2351, -222.3338) projected
  line L508 (-727.2351, -222.3338) -> (-727.6493, -222.2793) projected
  line L509 (-727.6493, -222.2793) -> (-728.0351, -222.1194) projected
  line L510 (-728.0351, -222.1194) -> (-728.3665, -221.8651) projected
  line L511 (-728.3665, -221.8651) -> (-728.6208, -221.5338) projected
  line L512 (-728.6208, -221.5338) -> (-728.7806, -221.1479) projected
  line L513 (-728.7806, -221.1479) -> (-728.8351, -220.7338) projected
  line L514 (-728.8351, -220.7338) -> (-728.7806, -220.3197) projected
  line L515 (-728.7806, -220.3197) -> (-728.6208, -219.9338) projected
  line L516 (-728.6208, -219.9338) -> (-728.3665, -219.6024) projected
  line L517 (-728.3665, -219.6024) -> (-728.0351, -219.3482) projected
  line L518 (-728.0351, -219.3482) -> (-727.6493, -219.1883) projected
  line L519 (-727.6493, -219.1883) -> (-727.2351, -219.1338) projected
  line L520 (-678.2351, -604.2338) -> (-611.7707, -670.6983) projected
  line L521 (-678.2351, -84.2338) -> (-678.2351, -604.2338) projected
  line L522 (-611.7707, -17.7693) -> (-678.2351, -84.2338) projected
  line L523 (-611.5131, -17.4555) -> (-611.7707, -17.7693) projected
  line L524 (-611.3217, -17.0974) -> (-611.5131, -17.4555) projected
  line L525 (-611.2039, -16.7089) -> (-611.3217, -17.0974) projected
  line L526 (-611.1641, -16.3049) -> (-611.2039, -16.7089) projected
  line L527 (-611.2039, -15.9008) -> (-611.1641, -16.3049) projected
  line L528 (-611.3217, -15.5123) -> (-611.2039, -15.9008) projected
  line L529 (-611.5131, -15.1542) -> (-611.3217, -15.5123) projected
  line L530 (-611.7707, -14.8404) -> (-611.5131, -15.1542) projected
  line L531 (-612.0845, -14.5828) -> (-611.7707, -14.8404) projected
  line L532 (-612.4426, -14.3915) -> (-612.0845, -14.5828) projected
  line L533 (-612.8311, -14.2736) -> (-612.4426, -14.3915) projected
  line L534 (-613.2351, -14.2338) -> (-612.8311, -14.2736) projected
  line L535 (-777.2351, -14.2338) -> (-613.2351, -14.2338) projected
  line L536 (-777.2351, -674.2338) -> (-777.2351, -14.2338) projected
  line L537 (-613.2351, -674.2338) -> (-777.2351, -674.2338) projected
  line L538 (-612.8311, -674.194) -> (-613.2351, -674.2338) projected
  line L539 (-612.4426, -674.0761) -> (-612.8311, -674.194) projected
  line L540 (-612.0845, -673.8848) -> (-612.4426, -674.0761) projected
  line L541 (-611.7707, -673.6272) -> (-612.0845, -673.8848) projected
  line L542 (-611.5131, -673.3134) -> (-611.7707, -673.6272) projected
  line L543 (-611.3217, -672.9553) -> (-611.5131, -673.3134) projected
  line L544 (-611.2039, -672.5668) -> (-611.3217, -672.9553) projected
  line L545 (-611.1641, -672.1627) -> (-611.2039, -672.5668) projected
  line L546 (-611.2039, -671.7587) -> (-611.1641, -672.1627) projected
  line L547 (-611.3217, -671.3702) -> (-611.2039, -671.7587) projected
  line L548 (-611.5131, -671.0121) -> (-611.3217, -671.3702) projected
  line L549 (-611.7707, -670.6983) -> (-611.5131, -671.0121) projected
  circle A0 centre (-638.2351, -29.2338) radius 2.4984
  circle A1 centre (-693.2351, -29.2338) radius 2.4984
  circle A2 centre (-763.2351, -29.2338) radius 2.4984
  circle A3 centre (-763.2351, -84.2338) radius 2.4984
  circle A4 centre (-693.2351, -84.2338) radius 2.4984
  circle A5 centre (-693.2351, -215.2838) radius 2.4984
  circle A6 centre (-763.2351, -215.2838) radius 2.4984
  circle A7 centre (-763.2351, -344.2338) radius 2.4984
  circle A8 centre (-763.2351, -473.1838) radius 2.4984
  circle A9 centre (-693.2351, -473.1838) radius 2.4984
  circle A10 centre (-693.2351, -344.2338) radius 2.4984
  circle A11 centre (-693.2351, -604.2338) radius 2.4984
  circle A12 centre (-763.2351, -604.2338) radius 2.4984
  circle A13 centre (-638.2351, -659.2338) radius 2.4984
  circle A14 centre (-763.2351, -659.2338) radius 2.4984
  circle A15 centre (-693.2351, -659.2338) radius 2.4984
  point P0 (-1999.0141, -29.8543)